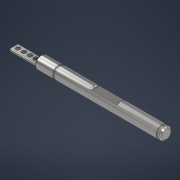
# Autodesk Inventor part: 023
Saved by Autodesk Inventor 2022 (Build 260153000, 153)
## iProperties
Created: 2021-11-21
Part Number: 023
Material: Stainless Steel, Austenitic
Document SubType Name: Modeling
Designer: vinicius.miguel
Density: 8 g/cm^3
Appearance: Semi-Polished
Author: vinicius.miguel
Autodesk Inventor part; units mm, degrees
ref_plane "YZ Plane" through (0, 0, 0) normal (1, 0, 0) x (0, 1, 0)
ref_plane "XY Plane" through (0, 0, 0) normal (0, 0, 1) x (1, 0, 0)
sketch "Sketch1" plane through (0, 0, 0) normal (1, 0, 0) x (0, 1, 0)
  circle A0 centre (0, 0) radius 4
  dimension "d0" = 8
  constraints: 1 centre point, 1 coincident
  measures "d0" diameter of A0
extrude "Extrusion1" add sketch "Sketch1" along normal blind 100
ref_plane "Work Plane1" through (0, 4, 0) normal (0, 1, 0) x (-1, 0, 0)
sketch "Sketch2" plane through (0, 4, 0) normal (0, 1, 0) x (-1, 0, 0)
  line L0 (0, 4.5363) -> (-18, 4.5363)
  line L1 (-18, 4.5363) -> (-18, -4.5363)
  line L2 (-18, -4.5363) -> (0, -4.5363)
  line L3 (0, -4.5363) -> (0, 4.5363)
  point P0 (0, 0)
  point P1 (0, 0)
  dimension "d3" = 18
  constraints: 8 end point, 2 midpoint, 2 parallel, 1 coincident, 1 horizontal, 1 perpendicular
  measures "d3" distance from line of L1 point (0, 0)
extrude "Extrusion2" cut sketch "Sketch2" against normal blind 4
sketch "Sketch3" plane through (0, 4, 0) normal (0, 1, 0) x (-1, 0, 0)
  line L0 (-55, 8.1957) -> (-72, 8.1957)
  line L1 (-72, 8.1957) -> (-72, -8.1957)
  line L2 (-72, -8.1957) -> (-55, -8.1957)
  line L3 (-55, -8.1957) -> (-55, 8.1957)
  point P0 (0, 0)
  point P1 (-55, 0)
  dimension "d6" = 17
  dimension "d38" = 55
  constraints: 8 end point, 2 parallel, 1 horizontal, 1 horizontal alignment, 1 midpoint, 1 perpendicular
  measures "d6" distance of L1.end L2.end
  measures "d38" distance from line of L3 point (0, 0)
extrude "Extrusion3" cut sketch "Sketch3" against normal blind 1
chamfer "Chamfer2" distance 0.5 angle 45 4 edges at (55, 3.7417, -1.4142) (55, 3.7417, 1.4142) (72, 3.7417, -1.4142) (72, 3.7417, 1.4142)
sketch "Sketch5" plane through (100, 0, 0) normal (1, 0, 0) x (0, 0, -1)
  circle A0 centre (0, 0) radius 3.5
  dimension "d22" = 7
  constraints: 1 centre point, 1 coincident
  measures "d22" diameter of A0
extrude "Extrusion4" add sketch "Sketch5" along normal blind 1
sketch "Sketch6" plane through (101, 0, 0) normal (1, 0, 0) x (0, 0, -1)
  circle A0 centre (0, 0) radius 4 projected
extrude "Extrusion5" add sketch "Sketch6" along normal blind 2
chamfer "Chamfer3" distance 1 angle 45 1 edges at (103, 0, 4)
sketch "Sketch7" plane through (0, 0, 0) normal (0, 1, 0) x (1, 0, 0)
  line L0 (18, -4) -> (18, 4) projected
  line L1 (0, 0) -> (3, 0)
  line L2 (3, 0) -> (7, 0)
  line L3 (7, 0) -> (11, 0)
  line L4 (11, 0) -> (15, 0)
  line L5 (15, 0) -> (18, 0)
  line L6 (18, 4) -> (18, -4) projected
  dimension "d53" = 4
  constraints: 10 end point, 6 collinear, 1 horizontal, 1 midpoint
  measures "d53" distance of L1.end L2.end
hole "Hole2" at (3, 0, 0) at (7, 0, 0) at (11, 0, 0) at (15, 0, 0) direction (0, -1, 0) diameter 2 end through all counterbore diameter 3 counterbore depth 2
sketch "Sketch8" plane through (0, 0, 0) normal (-1, 0, 0) x (0, 0, 1)
  arc A0 (4, 0) -> (-4, 0) centre (0, 0) ccw projected
  arc A1 (-4, 0) -> (4, 0) centre (0, 0) ccw projected
  arc A2 (3, 0) -> (-3, 0) centre (0, 0) ccw
  arc A3 (-3, 0) -> (3, 0) centre (0, 0) ccw
  dimension "d39" = 1
  constraints: 4 point on circle, 2 centre point, 1 other
  measures "d39" radial gap between concentric circles of A0 A2
extrude "Extrusion6" cut sketch "Sketch8" against normal up to surface (18 mm away)
chamfer "Chamfer4" distance 1 angle 45 1 edges at (18, -4, 0)
fillet "Fillet2" radius 0.5 4 edges at (0, -3, 0) (9, 0, 3) (0, 0, 0) (9, 0, -3)
sketch "Sketch9" plane through (0, 0, 0) normal (0, 0, 1) x (1, 0, 0)
  line L0 (1.5, 0) -> (4.5, 0) projected
  line L1 (4.5, -2) -> (1.5, -2) projected
  line L2 (5.5, 0) -> (8.5, 0) projected
  line L3 (8.5, -2) -> (5.5, -2) projected
  line L4 (9.5, 0) -> (12.5, 0) projected
  line L5 (12.5, -2) -> (9.5, -2) projected
  line L6 (13.5, 0) -> (16.5, 0) projected
  line L7 (16.5, -2) -> (13.5, -2) projected
  line L8 (1.5, -0.5) -> (1, -0.5)
  line L9 (1, -0.5) -> (1, -1)
  line L10 (1, -1) -> (1.5, -1)
  line L11 (1.5, -1) -> (1.5, -0.5)
  line L12 (3, 0) -> (3, -1.8019)
  point P0 (0, 0)
  dimension "d46" = 0.5
  dimension "d47" = 0.5
  dimension "d48" = 0.5
  constraints: 10 end point, 2 parallel, 1 horizontal, 1 midpoint, 1 perpendicular, 1 vertical, 1 vertical alignment
  measures "d46" distance of L10.end L8.start
  measures "d47" distance of L8.start L8.end
  measures "d48" distance from line of L0 L8.start
revolve "Revolution1" cut sketch "Sketch9" angle 360 about axis through (3, 0, 0) along (0, -1, 0)
pattern_linear "Rectangular Pattern1" count 4 spacing 4 along (1, 0, 0) of "Revolution1"
sketch "Sketch10" plane through (0, 0, 0) normal (0, 0, 1) x (1, 0, 0)
  line L0 (30.4, 4) -> (31.4, 4)
  line L1 (31.4, 4) -> (31.4, 3.5)
  line L2 (31.4, 3.5) -> (30.4, 3.5)
  line L3 (30.4, 3.5) -> (30.4, 4)
  line L4 (19, 4) -> (100, 4) projected
  line L5 (18, -0.6) -> (18, 3) projected
  line L6 (0, 0) -> (11.471, 0)
  dimension "d55" = 1
  dimension "d56" = 0.5
  dimension "d57" = 31.4
  constraints: 10 end point, 2 horizontal, 2 parallel, 1 perpendicular, 1 point on line
  measures "d55" distance of L1.end L2.end
  measures "d56" distance of L0.end L1.end
  measures "d57" distance from line of L1 L6.start
revolve "Revolution2" cut sketch "Sketch10" angle 360 about axis through (0, 0, 0) along (1, 0, 0)
body "Solid1"
